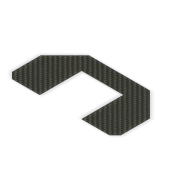
# Autodesk Inventor part: grip_tape
Saved by Autodesk Inventor 2020 (Build 240168000, 168)
## iProperties
Created: 2019-05-29
Part Number: grip_tape
Material: Generic
Document SubType Name: Modeling
Designer: chitl
Density: 1 g/cm^3
Appearance: Default
Author: chitl
Autodesk Inventor part; units mm, degrees
ref_plane "YZ Plane" through (0, 0, 0) normal (1, 0, 0) x (0, 1, 0)
ref_plane "XZ Plane" through (0, 0, 0) normal (0, 1, 0) x (-1, 0, 0)
ref_plane "XY Plane" through (0, 0, 0) normal (0, 0, 1) x (1, 0, 0)
sketch "Sketch1" plane through (0, 0, 0) normal (0, 1, 0) x (-1, 0, 0)
  line L0 (25.2755, 50.8) -> (25.2755, -12.7)
  line L1 (25.2755, -12.7) -> (-25.5245, -12.7)
  line L2 (-25.5245, -12.7) -> (-25.5245, 50.8)
  line L3 (-25.5245, 50.8) -> (-76.2, 50.8)
  line L4 (-76.2, 50.8) -> (-88.9, 38.1)
  line L5 (-88.9, 38.1) -> (-88.9, -10.8962)
  line L6 (-88.9, -10.8962) -> (-48.9962, -50.8)
  line L7 (-48.9962, -50.8) -> (48.9962, -50.8)
  line L8 (48.9962, -50.8) -> (88.9, -10.8962)
  line L9 (88.9, -10.8962) -> (88.9, 38.1)
  line L10 (88.9, 38.1) -> (76.2, 50.8)
  line L11 (76.2, 50.8) -> (25.2755, 50.8)
  line L12 (82.55, -8.2659) -> (46.3659, -44.45)
  line L13 (46.3659, -44.45) -> (-46.3659, -44.45)
  line L14 (-46.3659, -44.45) -> (-82.55, -8.2659)
  line L15 (-82.55, -8.2659) -> (-82.55, 35.4697)
  line L16 (-82.55, 35.4697) -> (-73.5697, 44.45)
  line L17 (-73.5697, 44.45) -> (-31.8745, 44.45)
  line L18 (-31.8745, 44.45) -> (-31.8745, -19.05)
  line L19 (-31.8745, -19.05) -> (31.6255, -19.05)
  line L20 (31.6255, -19.05) -> (31.6255, 44.45)
  line L21 (31.6255, 44.45) -> (73.5697, 44.45)
  line L22 (73.5697, 44.45) -> (82.55, 35.4697)
  line L23 (82.55, 35.4697) -> (82.55, -8.2659)
  point P0 (0, 0)
  point P1 (82.55, -8.2659)
  constraints: 48 end point
extrude "Extrusion1" add sketch "Sketch1" along normal blind 0.1 contours L12 L13 L14 L15 L16 L17 L18 L19 L20 L21 L22 L23
body "Solid1"
